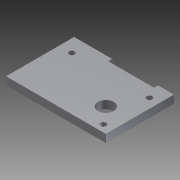
# Autodesk Inventor part: carro x lado motor pieza 2parte 2-2
Saved by Autodesk Inventor 2012 (Build 160160000, 160)
## iProperties
Created: 2014-12-17
Part Number: carro x lado motor pieza 2parte 2-2
Material: Default
Document SubType Name: Modeling
Designer: PRINCIPAL
Density: 1 g/cm^3
Author: PRINCIPAL
Autodesk Inventor part; units mm, degrees
ref_plane "YZ Plane" through (0, 0, 0) normal (1, 0, 0) x (0, 1, 0)
ref_plane "XZ Plane" through (0, 0, 0) normal (0, 1, 0) x (-1, 0, 0)
ref_plane "XY Plane" through (0, 0, 0) normal (0, 0, 1) x (1, 0, 0)
sketch "Boceto1" plane through (0, 0, 0) normal (0, 0, 1) x (1, 0, 0)
  line L0 (-12.1173, 0.2988) -> (-22.1173, 0.2988)
  line L1 (-22.1173, 0.2988) -> (-22.1173, -2.2012)
  line L2 (-22.1173, -2.2012) -> (-51.1173, -2.2012)
  line L3 (-51.1173, -2.2012) -> (-51.1173, 0.2988)
  line L4 (-51.1173, 0.2988) -> (-75.1173, 0.2988)
  line L5 (-75.1173, 0.2988) -> (-75.1173, -42.7012)
  line L6 (-75.1173, -42.7012) -> (-12.1173, -42.7012)
  line L7 (-12.1173, -42.7012) -> (-12.1173, 0.2988)
  circle A0 centre (-18.1173, -9.2012) radius 1.75
  circle A1 centre (-67.1173, -9.2012) radius 1.75
  circle A2 centre (-18.1173, -38.2012) radius 1.7568
  circle A3 centre (-27.1173, -27.7012) radius 5
  point P0 (0, 0)
  constraints: 16 end point, 4 centre point
extrude "Extrusión1" add sketch "Boceto1" along normal blind 5
